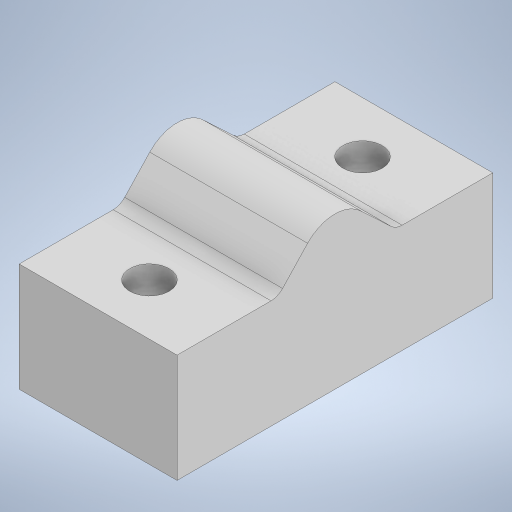
# Autodesk Inventor part: linac_lower_ax_mount
Saved by Autodesk Inventor 2024 (Build 280153000, 153)
## iProperties
Created: 2025-12-25
Part Number: linac_lower_ax_mount
Material: Generic
Document SubType Name: Modeling
Designer: schar
Density: 1 g/cm^3
Appearance: Default
Author: schar
Autodesk Inventor part; units mm, degrees
ref_plane "YZ Plane" through (0, 0, 0) normal (1, 0, 0) x (0, 1, 0)
ref_plane "XZ Plane" through (0, 0, 0) normal (0, 1, 0) x (-1, 0, 0)
ref_plane "XY Plane" through (0, 0, 0) normal (0, 0, 1) x (1, 0, 0)
sketch "Sketch1" plane through (0, 0, 0) normal (1, 0, 0) x (0, 1, 0)
  circle A0 centre (0, 0) radius 3.25
  circle A1 centre (0, 0) radius 4.75
  line L0 (-4.75, 0) -> (-4.75, -20)
  line L1 (-4.75, 0) -> (-4.75, 20)
  line L2 (-4.75, 20) -> (-0.75, 20)
  line L3 (-0.75, 20) -> (-0.75, 4.6904)
  line L4 (-0.75, -4.6904) -> (-0.75, -20)
  line L5 (-4.75, -20) -> (-0.75, -20)
  line L6 (3.2538, 3.4605) -> (-0.75, 7.2252)
  line L7 (3.2538, -3.4605) -> (-0.75, -7.7187)
  dimension "d0" = 6.5
  dimension "d1" = 9.5
  dimension "d2" = 20
  dimension "d3" = 20
  dimension "d4" = 4
  constraints: 16 end point, 5 point on circle, 4 perpendicular, 3 tangent, 3 vertical, 2 centre point, 2 coincident, 2 point on line
  measures "d0" diameter of A0
  measures "d1" diameter of A1
  measures "d2" distance of L0.start L0.end
  measures "d3" distance of L0.start L1.end
  measures "d4" distance of L1.end L2.end
extrude "Extrusion1" add sketch "Sketch1" along normal blind 20
sketch "Sketch3" plane through (0, -0.75, 20) normal (0, 1, 0) x (1, 0, 0)
  line L0 (0, 0) -> (0, 40) projected
  line L1 (0, 0) -> (10, 0)
  line L2 (0, 0) -> (20, 0) projected
  line L3 (10, 0) -> (10, 6.5)
  line L4 (0, 40) -> (20, 40) projected
  line L5 (0, 40) -> (10, 40)
  line L6 (10, 40) -> (10, 33.5)
  circle A0 centre (10, 6.5) radius 2.5
  circle A1 centre (10, 33.5) radius 2.5
  point P0 (0, 20)
  dimension "d7" = 6.5
  dimension "d8" = 6.5
  dimension "d9" = 5
  dimension "d10" = 5
  constraints: 8 end point, 2 centre point, 2 coincident, 2 midpoint, 2 perpendicular
  measures "d7" distance of L1.end L3.end
  measures "d8" distance of L5.end L6.end
  measures "d9" diameter of A0
  measures "d10" diameter of A1
extrude "Extrusion2" cut sketch "Sketch3" against normal blind 20
fillet "Fillet1" radius 2 2 edges at (10, -0.75, 7.2252) (10, -0.75, -7.7187)
sketch "Sketch4" plane through (20, 0, 0) normal (1, 0, 0) x (0, 0, -1)
  circle A0 centre (0, 0) radius 3.25
  constraints: 1 centre point, 1 coincident
extrude "Extrusion3" add sketch "Sketch4" against normal blind 10
sketch "Sketch5" plane through (0, -4.75, -20) normal (0, -1, 0) x (1, 0, 0)
  line L0 (0, 0) -> (20, 0) projected
  line L1 (20, 40) -> (20, 0) projected
  line L2 (0, 0) -> (20, 0)
  line L3 (20, 0) -> (20, 40)
  line L4 (20, 40) -> (0, 40)
  line L5 (0, 40) -> (0, 0)
  circle A0 centre (10, 6.5) radius 2.5 projected
  circle A1 centre (10, 6.5) radius 2.5
  circle A2 centre (10, 33.5) radius 2.5 projected
  circle A3 centre (10, 33.5) radius 2.5
  point P0 (0, 20)
  constraints: 8 end point, 2 centre point, 2 coincident, 2 parallel, 1 horizontal, 1 perpendicular
extrude "Extrusion4" add sketch "Sketch5" along normal blind 9.75
body "Solid1"
